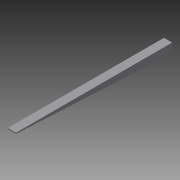
# Autodesk Inventor part: 1x1 lengthwise right
Saved by Autodesk Inventor 2015 SP1 (Build 190203100, 203)
## iProperties
Created: 2015-01-16
Part Number: 1x1 lengthwise right
Material: Generic
Document SubType Name: Modeling
Designer: Jarod
Density: 1 g/cm^3
Appearance: Default
Author: Jarod
Autodesk Inventor part; units mm, degrees
ref_plane "YZ Plane" through (0, 0, 0) normal (1, 0, 0) x (0, 1, 0)
ref_plane "XZ Plane" through (0, 0, 0) normal (0, 1, 0) x (-1, 0, 0)
ref_plane "XY Plane" through (0, 0, 0) normal (0, 0, 1) x (1, 0, 0)
sketch "Sketch1" plane through (0, 0, 0) normal (0, 0, 1) x (1, 0, 0)
  line L0 (0, 0) -> (-25.4, 0)
  line L1 (-25.4, 0) -> (-25.4, -3.175)
  line L2 (-25.4, -3.175) -> (0, -3.175)
  line L3 (0, -3.175) -> (0, 0)
  line L4 (0, 0) -> (-3.175, 0)
  line L5 (-3.175, 0) -> (-3.175, -25.4)
  line L6 (-3.175, -25.4) -> (0, -25.4)
  line L7 (0, -25.4) -> (0, 0)
  dimension "d0" = 25.4
  dimension "d1" = 3.175
  dimension "d2" = 3.175
  dimension "d3" = 25.4
  constraints: 16 end point, 4 parallel, 2 horizontal, 2 perpendicular
  measures "d0" distance of L2.end L1.end
  measures "d1" distance of L1.end L0.end
  measures "d2" distance of L6.end L5.end
  measures "d3" distance of L5.end L4.end
extrude "Extrusion1" add sketch "Sketch1" along normal blind 431.8
sketch "Sketch2" plane through (0, -25.4, 0) normal (1, 0, 0) x (0, 0, -1)
  line L0 (0, 0) -> (0, 25.4) projected
  line L1 (0, 25.4) -> (-431.8, 25.4) projected
  line L2 (-431.8, 0) -> (-431.8, 25.4) projected
  line L3 (0, 0) -> (-431.8, 0) projected
  line L4 (0, 0) -> (-50.8, 0) construction
  line L5 (0, 0) -> (-431.8, 0) construction
  line L6 (-431.8, 25.4) -> (-431.8, 22.225) construction
  line L7 (-431.8, 22.225) -> (-50.8, 0)
  line L8 (-431.8, 22.225) -> (-431.8, 0)
  line L9 (-431.8, 0) -> (-50.8, 0)
  dimension "d6" = 50.8
  dimension "d7" = 3.175
  constraints: 10 end point, 2 perpendicular, 2 point on line
  measures "d6" distance of L0.start L4.end
  measures "d7" distance of L1.end L6.end
extrude "Extrusion2" cut sketch "Sketch2" against normal blind 25.4 contours L3 L2 L7
sketch "Sketch3" plane through (0, -25.4, 0) normal (1, 0, 0) x (0, 0, -1)
  line L0 (-431.8, 22.225) -> (-50.8, 0) projected
  line L1 (0, 0) -> (-50.8, 0) projected
  line L2 (0, 0) -> (0, 25.4) projected
  line L3 (0, 25.4) -> (-431.8, 25.4) projected
  line L4 (-431.8, 22.225) -> (-431.8, 25.4) projected
  point P0 (-38.1, 12.7)
  point P1 (-12.7, 12.7)
  dimension "d10" = 12.7
  dimension "d11" = 12.7
  dimension "d12" = 38.1
  dimension "d13" = 12.7
  measures "d10" distance from line of L3 point (-12.7, 12.7)
  measures "d11" distance from line of L2 point (-12.7, 12.7)
  measures "d12" distance from line of L2 point (-38.1, 12.7)
  measures "d13" distance from line of L3 point (-38.1, 12.7)
hole "Hole1" at (0, -12.7, 38.1) at (0, -12.7, 12.7) direction (-1, 0, 0) diameter 6.35 end through all
sketch "Sketch4" plane through (-25.4, 0, 0) normal (0, 1, 0) x (1, 0, 0)
  line L0 (25.4, 0) -> (0, 0) projected
  line L1 (0, 0) -> (0, -431.8) projected
  line L2 (25.4, -431.8) -> (0, -431.8) projected
  line L3 (25.4, 0) -> (25.4, -431.8) projected
  point P0 (12.7, -15.875)
  point P1 (12.7, -206.375)
  point P2 (12.7, -409.575)
  dimension "d21" = 12.7
  dimension "d22" = 12.7
  dimension "d23" = 12.7
  dimension "d24" = 15.875
  dimension "d25" = 206.375
  dimension "d26" = 22.225
  measures "d21" distance from line of L3 point (12.7, -15.875)
  measures "d22" distance from line of point (12.7, -206.375) L3
  measures "d23" distance from line of L3 point (12.7, -409.575)
  measures "d24" distance from line of L0 point (12.7, -15.875)
  measures "d25" distance from line of L0 point (12.7, -206.375)
  measures "d26" distance from line of L2 point (12.7, -409.575)
hole "Hole2" at (-12.7, 0, 15.875) at (-12.7, 0, 206.375) at (-12.7, 0, 409.575) direction (0, -1, 0) diameter 6.35 end through all
body "Solid1"
